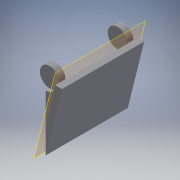
# Autodesk Inventor part: NASA-20-ARM-SH-01
Saved by Autodesk Inventor 2019 (Build 230136000, 136)
## iProperties
Created: 2019-09-09
Part Number: NASA-20-ARM-SH-01
Material: Generic
Document SubType Name: Modeling
Designer: Rick Szalay
Density: 1 g/cm^3
Appearance: Default
Author: Rick Szalay
Autodesk Inventor part; units mm, degrees
ref_plane "YZ Plane" through (0, 0, 0) normal (1, 0, 0) x (0, 1, 0)
ref_plane "XZ Plane" through (0, 0, 0) normal (0, 1, 0) x (-1, 0, 0)
ref_plane "XY Plane" through (0, 0, 0) normal (0, 0, 1) x (1, 0, 0)
sketch "Sketch1" plane through (0, 0, 0) normal (0, 0, 1) x (1, 0, 0)
  line L0 (0, 50.8) -> (0, -50.8)
  line L1 (0, -50.8) -> (25.4, 50.8)
  line L2 (25.4, 50.8) -> (0, 50.8)
  point P0 (0, 0)
  point P1 (0, 0)
  dimension "d0" = 101.6
  dimension "d2" = 25.4
  constraints: 6 end point, 1 coincident, 1 horizontal, 1 midpoint, 1 vertical
  measures "d0" distance of L0.start L0.end
  measures "d2" distance of L1.end L0.start
extrude "Extrusion1" add sketch "Sketch1" along normal mid plane 127
sketch "Sketch2" plane through (0, 0, 0) normal (0, 0, 1) x (1, 0, 0)
  line L0 (0, 50.8) -> (0, -50.8) projected
  circle A0 centre (0, 50.8) radius 15
  point P0 (0, 0)
  dimension "d5" = 30
  constraints: 1 centre point
  measures "d5" diameter of A0
extrude "Extrusion2" add sketch "Sketch2" along normal mid plane 114.3
sketch "Sketch3" plane through (0, 0, 63.5) normal (0, 0, 1) x (1, 0, 0)
  line L0 (0, 50.8) -> (0, -50.8) projected
  line L1 (0, 50.8) -> (25.4, 50.8) projected
  arc A0 (0, 35.8) -> (15, 50.8) centre (0, 50.8) ccw
  arc A1 (15, 50.8) -> (0, 35.8) centre (0, 50.8) ccw projected
  point P0 (0, 0)
  constraints: 2 concentric, 2 point on circle, 2 point on line, 1 centre point
extrude "Extrusion3" cut sketch "Sketch3" against normal up to surface (6.35 mm away) contours L1 A0 L0
mirror "Mirror1" about plane through (0, 0, 0) normal (0, 0, 1) of "Extrusion3"
ref_plane "Work Plane1" through (14.5521, 47.162, 0) normal (0.9701425, -0.2425356, 0) x (0.2425356, 0.9701425, 0)
sketch "Sketch4" plane through (14.5521, 47.162, 0) normal (0.9701425, -0.2425356, 0) x (0.2425356, 0.9701425, 0)
  line L0 (15, -57.15) -> (15, 57.15) projected
  line L1 (15, 47.625) -> (-14.5521, 47.625)
  line L2 (-14.5521, 47.625) -> (-98.5665, 57.15)
  line L3 (-98.5665, -63.5) -> (-98.5665, 63.5) projected
  line L4 (15, 0) -> (-98.5665, 0) construction
  line L5 (15, 57.15) -> (-15, 57.15) construction
  line L6 (-15, -57.15) -> (-15, 57.15) construction
  line L7 (-14.5521, 57.15) -> (-14.5521, -57.15) construction
  line L8 (15, -47.625) -> (-14.5521, -47.625)
  line L9 (-14.5521, -47.625) -> (-98.5665, -57.15)
  line L10 (15, 47.625) -> (15, -47.625)
  line L11 (-98.5665, 57.15) -> (-98.5665, -57.15)
  point P0 (-49.2832, 0)
  point P1 (3.638, 57.15)
  dimension "d10" = 6.35
  dimension "d11" = 9.525
  constraints: 14 end point, 3 point on line, 3 symmetric about line, 2 midpoint, 1 horizontal, 1 parallel, 1 perpendicular
  measures "d10" distance of L2.end L3.end
  measures "d11" distance between parallel lines of L5 L1
extrude "Extrusion4" cut sketch "Sketch4" against normal through all
body "Solid1"
